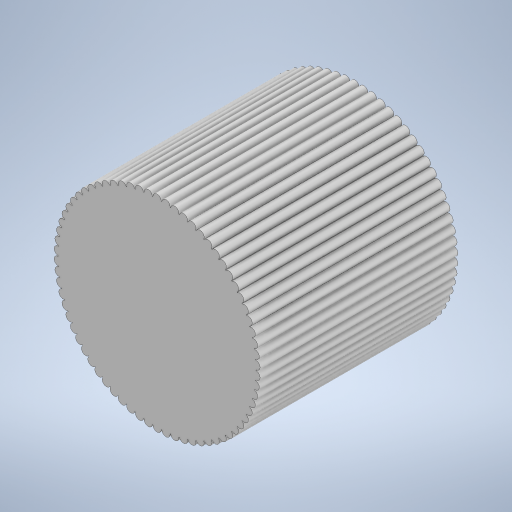
# Autodesk Inventor part: ex_tank_inter
Saved by Autodesk Inventor 2024 (Build 280153000, 153)
## iProperties
Created: 2023-06-07
Part Number: ex_tank_inter
Material: Generic
Document SubType Name: Modeling
Designer: tamiz
Density: 1 g/cm^3
Appearance: Default
Author: tamiz
Autodesk Inventor part; units mm, degrees
ref_plane "YZ Plane" through (0, 0, 0) normal (1, 0, 0) x (0, 1, 0)
ref_plane "XZ Plane" through (0, 0, 0) normal (0, 1, 0) x (-1, 0, 0)
ref_plane "XY Plane" through (0, 0, 0) normal (0, 0, 1) x (1, 0, 0)
sketch "Sketch1" plane through (0, 0, 0) normal (0, 0, 1) x (1, 0, 0)
  circle A0 centre (0, 0) radius 5334
  dimension "d0" = 10668
  constraints: 1 centre point, 1 coincident
  measures "d0" diameter of A0
extrude "Extrusion1" add sketch "Sketch1" against normal blind 10668
sketch "Sketch2" plane through (0, 0, 0) normal (0, 0, 1) x (1, 0, 0)
  circle A0 centre (0, 0) radius 4876.8
  constraints: 1 centre point, 1 coincident
extrude "Extrusion4" cut sketch "Sketch2" against normal blind 10210.8
sketch "Sketch5" plane through (0, 0, 0) normal (0, 0, 1) x (1, 0, 0)
  circle A0 centre (0, 0) radius 5334
  constraints: 1 centre point, 1 coincident
extrude "Extrusion5" add sketch "Sketch5" against normal blind 457.2
sketch "Sketch6" plane through (0, 0, 0) normal (0, 0, 1) x (1, 0, 0)
  circle A0 centre (0, 0) radius 5334 projected
  circle A1 centre (0, 5334) radius 228.6
  point P0 (228.5475, 5329.1014)
  point P1 (-228.5475, 5329.1014)
  dimension "d17" = 457.2
  constraints: 1 centre point, 2 other
  measures "d17" diameter of A1
extrude "Extrusion6" add sketch "Sketch6" against normal blind 10668 contours A0 A1 picked at (-0.8165, 5410.065)
pattern_circular "Circular Pattern1" count 70 over 360 about axis through (0, 0, -10) along (0, 0, 1) of "Extrusion6"
body "Solid1"
